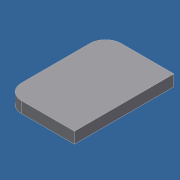
# Autodesk Inventor part: P1704_018_hautManette
Saved by Autodesk Inventor 2019 (Build 230136000, 136)
## iProperties
Created: 2019-05-28
Part Number: P1704_018_hautManette
Project: Nom Projet
Material: .
Description: Nom pièce
Document SubType Name: Modeling
Designer: Adel.KAHRIMANOVIC
Authority: brut Ø
Density: 0.001 g/cm^3
Appearance: Par défaut
Author: Adel.KAHRIMANOVIC
Material number: ---
Autodesk Inventor part; units mm, degrees
ref_plane "Plan YZ" through (0, 0, 0) normal (1, 0, 0) x (0, 1, 0)
ref_plane "Plan XZ" through (0, 0, 0) normal (0, 1, 0) x (-1, 0, 0)
ref_plane "Plan XY" through (0, 0, 0) normal (0, 0, 1) x (1, 0, 0)
sketch "Esquisse1" plane through (0, 0, 0) normal (0, 0, 1) x (1, 0, 0)
  line L0 (55, 80) -> (55, -80)
  line L1 (-55, -80) -> (-55, 80)
  line L2 (-55, 80) -> (55, -80) construction
  line L3 (55, 80) -> (-55, -80) construction
  line L4 (0, 0) -> (-55, 0) construction
  arc A0 (-55, -55) -> (-30, -80) centre (-30, -55) ccw
  line L5 (-30, -80) -> (55, -80)
  line L6 (-30, -80) -> (-30, -55) construction
  line L7 (55, 80) -> (-30, 80)
  arc A1 (-30, 80) -> (-55, 55) centre (-30, 55) ccw
  line L8 (-30, 55) -> (-30, 80) construction
  line L9 (-83.2132, 0) -> (78.0355, 0) projected
  line L10 (0, -119.2487) -> (0, 119.2487) projected
  dimension "d2" = 160
  dimension "d3" = 110
  dimension "d4" = 25
  dimension "d5" = 25
  constraints: 18 end point, 4 midpoint, 4 point on circle, 3 horizontal, 2 centre point, 2 parallel, 2 point on line, 2 tangent, 2 vertical, 1 collinear, 1 perpendicular
  measures "d2" distance of L0.start L0.end
  measures "d3" distance of L0.end L1.start
  measures "d4" distance of L5.start L6.end
  measures "d5" distance of L8.start L7.end
extrude "Extrusion1" add sketch "Esquisse1" along normal blind 20
sketch "Esquisse6" plane through (0, 0, 0) normal (0, 0, -1) x (-1, 0, 0)
  line L0 (-52.5, 77.5) -> (-52.5, -77.5)
  line L1 (-52.5, -77.5) -> (30, -77.5)
  line L2 (-52.5, 77.5) -> (30, 77.5)
  arc A0 (52.5, 55) -> (30, 77.5) centre (30, 55) ccw
  line L3 (52.5, 55) -> (52.5, -55)
  arc A1 (30, -77.5) -> (52.5, -55) centre (30, -55) ccw
  line L4 (-55, 80) -> (30, 80) projected
  line L5 (-55, -80) -> (-55, 80) projected
  line L6 (30, -80) -> (-55, -80) projected
  line L7 (55, 55) -> (55, -55) projected
  line L8 (30, -239.7653) -> (30, 84.7653) construction
  arc A2 (55, 55) -> (30, 80) centre (30, 55) ccw projected
  line L9 (-55, -80) -> (-55, 80) projected
  line L10 (30, -80) -> (-55, -80) projected
  arc A3 (30, -80) -> (55, -55) centre (30, -55) ccw projected
  line L11 (55, 55) -> (55, -55) projected
  arc A4 (55, 55) -> (30, 80) centre (30, 55) ccw projected
  line L12 (-55, 80) -> (30, 80) projected
  point P0 (0, 0)
  dimension "d8" = 2.5
  dimension "d9" = 2.5
  dimension "d10" = 2.5
  dimension "d11" = 2.5
  constraints: 10 end point, 4 point on circle, 4 tangent, 3 vertical, 2 centre point, 2 point on line, 1 horizontal, 1 midpoint, 1 perpendicular
  measures "d8" distance between parallel lines of L4 L2
  measures "d9" distance between parallel lines of L5 L0
  measures "d10" distance between parallel lines of L6 L1
  measures "d11" distance between parallel lines of L7 L3
extrude "Extrusion2" cut sketch "Esquisse6" against normal blind 2
sketch "Esquisse7" plane through (0, 0, 0) normal (0, 0, -1) x (-1, 0, 0)
  line L0 (-50, 75) -> (-50, -75)
  line L1 (-50, -75) -> (30, -75)
  line L2 (50, 55) -> (50, -55)
  line L3 (-50, 75) -> (30, 75)
  arc A0 (50, 55) -> (30, 75) centre (30, 55) ccw
  arc A1 (30, -75) -> (50, -55) centre (30, -55) ccw
  line L4 (30, 77.5) -> (-52.5, 77.5) projected
  line L5 (-52.5, 77.5) -> (-52.5, -77.5) projected
  line L6 (-52.5, -77.5) -> (30, -77.5) projected
  line L7 (52.5, -55) -> (52.5, 55) projected
  line L8 (30, 77.5) -> (30, 105.4816) construction
  point P0 (0, 0)
  dimension "d14" = 2.5
  dimension "d15" = 2.5
  dimension "d16" = 2.5
  dimension "d17" = 2.5
  constraints: 10 end point, 4 point on circle, 4 tangent, 3 vertical, 2 centre point, 2 point on line, 1 horizontal, 1 perpendicular
  measures "d14" distance between parallel lines of L3 L4
  measures "d15" distance between parallel lines of L5 L0
  measures "d16" distance between parallel lines of L6 L1
  measures "d17" distance between parallel lines of L7 L2
extrude "Extrusion3" cut sketch "Esquisse7" against normal blind 18
